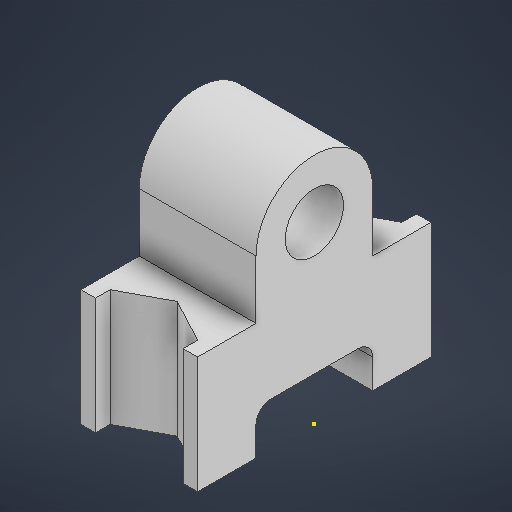
# Autodesk Inventor part: Peça3
Saved by Autodesk Inventor 2027.1 (Build 311270010, 270A)
## iProperties
Created: 2026-09-24
Part Number: Peça3
Material: Genérico
Document SubType Name: Modeling
Designer: carlo
Density: 1 g/cm^3
Appearance: Padrão
Author: carlo
Autodesk Inventor part; units mm, degrees
ref_plane "YZ Plane" through (0, 0, 0) normal (1, 0, 0) x (0, 1, 0)
ref_plane "XZ Plane" through (0, 0, 0) normal (0, 1, 0) x (-1, 0, 0)
ref_plane "XY Plane" through (0, 0, 0) normal (0, 0, 1) x (1, 0, 0)
sketch "Esboço1" plane through (0, 0, 0) normal (0, 1, 0) x (-1, 0, 0)
  line L0 (20, 40) -> (-20, 40)
  line L1 (-20, 40) -> (-20, -40)
  line L2 (-20, -40) -> (20, -40)
  line L3 (20, -40) -> (20, 40)
  line L4 (20, 40) -> (-20, -40) construction
  line L5 (-20, 40) -> (20, -40) construction
  point P0 (0, 0)
  dimension "d0" = 40
  dimension "d1" = 80
  constraints: 12 end point, 2 midpoint, 2 parallel, 1 horizontal, 1 perpendicular
  measures "d0" distance of L2.end L1.end
  measures "d1" distance of L1.end L0.end
extrude "Extrusão1" add sketch "Esboço1" along normal blind 80
sketch "Esboço2" plane through (20, 0, 40) normal (1, 0, 0) x (0, 0, -1)
  line L0 (0, 80) -> (80, 80) projected
  line L1 (0, 80) -> (20, 80)
  line L2 (20, 80) -> (20, 40)
  line L3 (20, 40) -> (0, 40)
  line L4 (0, 40) -> (0, 80)
  line L5 (80, 80) -> (60, 80)
  line L6 (60, 80) -> (60, 40)
  line L7 (60, 40) -> (80, 40)
  line L8 (80, 40) -> (80, 80)
  line L9 (0, 0) -> (80, 0) projected
  point P0 (40, 0)
  point P1 (60, 60)
  point P2 (20, 80)
  dimension "d4" = 40
  dimension "d5" = 20
  dimension "d6" = 20
  constraints: 16 end point, 4 parallel, 2 horizontal, 2 perpendicular, 1 midpoint, 1 point on line
  measures "d4" distance between parallel lines of L3 L9
  measures "d5" distance from line of point (60, 60) L8
  measures "d6" distance between parallel lines of L4 L2
extrude "Extrusão2" cut sketch "Esboço2" against normal blind 80
fillet "Arredondamento1" radius 20 2 edges at (0, 80, 20) (0, 80, -20)
sketch "Esboço3" plane through (20, 0, 40) normal (1, 0, 0) x (0, 0, -1)
  arc A0 (60, 60) -> (20, 60) centre (40, 60) ccw projected
  point P0 (40, 0)
  constraints: 1 coincident
hole "Furo1" at (20, 60, 0) direction (-1, 0, 0) diameter 20 end through all
sketch "Esboço4" plane through (20, 40, 40) normal (0, 1, 0) x (1, 0, 0)
  line L0 (0, 0) -> (0, 80) projected
  line L1 (0, 0) -> (-5, 0)
  line L2 (-40, 0) -> (0, 0) projected
  line L3 (-5, 0) -> (-5, 5)
  line L4 (-40, 0) -> (-35, 0)
  line L5 (-35, 0) -> (-35, 5)
  line L6 (-35, 0) -> (-20, 0) construction
  line L7 (-20, 0) -> (-20, 13) construction
  line L8 (-35, 5) -> (-20, 13)
  line L9 (-20, 13) -> (-5, 5)
  point P0 (-20, 40)
  dimension "d17" = 5
  dimension "d18" = 5
  dimension "d19" = 5
  dimension "d20" = 15
  dimension "d21" = 13
  constraints: 16 end point, 3 perpendicular, 2 point on line, 1 midpoint
  measures "d17" distance of L0.start L1.end
  measures "d18" distance of L1.end L3.end
  measures "d19" distance of L2.start L4.end
  measures "d20" distance of L4.end L6.end
  measures "d21" distance of L6.end L7.end
extrude "Extrusão3" cut sketch "Esboço4" against normal blind 80
mirror "Espelhar1" about plane through (0, 0, 0) normal (0, 0, 1) of "Extrusão3"
sketch "Esboço5" plane through (20, 0, 40) normal (1, 0, 0) x (0, 0, -1)
  point P0 (40, 0)
sketch "Esboço6" plane through (20, 0, 40) normal (1, 0, 0) x (0, 0, -1)
  line L0 (0, 0) -> (0, 40) construction
  line L1 (0, 0) -> (20, 0) construction
  line L2 (0, 0) -> (80, 0) construction
  line L3 (20, 0) -> (20, 15)
  line L4 (20, 15) -> (60, 15)
  line L5 (60, 15) -> (60, 0)
  line L6 (60, 0) -> (20, 0)
  point P0 (40, 0)
  dimension "d24" = 20
  dimension "d25" = 15
  dimension "d26" = 40
  constraints: 10 end point, 2 parallel, 2 perpendicular, 1 point on line
  measures "d24" distance of L0.start L1.end
  measures "d25" distance of L1.end L3.end
  measures "d26" distance of L3.end L4.end
extrude "Extrusão4" cut sketch "Esboço6" against normal blind 80
fillet "Arredondamento2" radius 5 2 edges at (0, 15, -20) (0, 15, 20)
